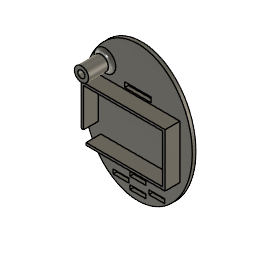
Panel2 (Autodesk Fusion 360 design; units mm, degrees)
part number: 2026-05-24-13-53-39-480
Autodesk Fusion 360 part; units mm, degrees
sketch "Sketch1" plane through (0, 0, 0) normal (0, 1, 0) x (1, 0, 0)
  ellipse E0 centre (0, 0) end of major axis (0, 27.5) minor radius 22
  line L0 (0, -27.5) -> (0, 27.5) construction
  line L1 (22, 0) -> (-22, 0) construction
  dimension "d1" = 44
  dimension "d2" = 55
  constraint coincident E0 L0.start
  constraint coincident E0 L0.end
  constraint coincident E0 L1.start
  constraint coincident E0 L1.end
  constraint coincident E0.centre origin
  constraint vertical L0
  measures "d2" distance of E0
extrude "Extrude1" add sketch "Sketch1" along normal blind 1.5
sketch "Sketch2" plane through (0, 0, 0) normal (0, -1, 0) x (1, 0, 0)
  ellipse E0 centre (0, 0) end of major axis (0, -27.5) minor radius 22
  line L0 (-5.35, 11.5) -> (5.35, 11.5)
  line L1 (5.35, 11.5) -> (5.35, 9.5)
  line L2 (5.35, 9.5) -> (-5.35, 9.5)
  line L3 (-5.35, 9.5) -> (-5.35, 11.5)
  point P0 (0, 27.5)
  dimension "d5" = 10.7
  dimension "d6" = 2
  dimension "d7" = 16
  constraint horizontal L0
  constraint vertical L1
  constraint horizontal L2
  constraint vertical L3
  constraint coincident E0 P0
  measures "d5" distance of L1.end L2.end
  measures "d6" distance of L0.start L2.end
  measures "d7" distance of L0 P0
extrude "Extrude2" cut sketch "Sketch2" against normal blind 10 contours L0 L1 L2 L3
sketch "Sketch3" plane through (0, 0, 0) normal (0, -1, 0) x (1, 0, 0)
  line L0 (5.35, 11.5) -> (5.35, 9.5)
  line L1 (5.35, 9.5) -> (-5.35, 9.5)
  line L2 (-5.35, 9.5) -> (-5.35, 11.5)
  line L3 (-5.35, 11.5) -> (5.35, 11.5)
  ellipse E0 centre (0, 0) end of major axis (0, -27.5) minor radius 22
  circle A0 centre (-13.3446, 14.9401) radius 1.45
  circle A1 centre (-13.3446, 14.9401) radius 2.9
  dimension "d10" = 2.9
  dimension "d11" = 5.8
  constraint concentric A0 A1
  measures "d10" diameter of A0
  measures "d11" diameter of A1
extrude "Extrude3" add sketch "Sketch3" along normal blind 9.5 contours A1
fillet "Fillet1" radius 1.5 1 edges at (-16.0483, 0, 15.9888)
sketch "Sketch4" plane through (0, 0, 0) normal (0, -1, 0) x (1, 0, 0)
  line L0 (5.35, 11.5) -> (5.35, 9.5)
  line L1 (5.35, 9.5) -> (-5.35, 9.5)
  line L2 (-5.35, 9.5) -> (-5.35, 11.5)
  line L3 (-5.35, 11.5) -> (5.35, 11.5)
  line L4 (-16, 7.9) -> (16, 7.9)
  line L5 (16, 7.9) -> (16, -11.6)
  line L6 (16, -11.6) -> (-16, -11.6)
  line L7 (-16, -11.6) -> (-16, 7.9)
  line L8 (-17, 8.9) -> (17, 8.9)
  line L9 (17, 8.9) -> (17, -12.6)
  line L10 (17, -12.6) -> (-17, -12.6)
  line L11 (-17, -12.6) -> (-17, 8.9)
  ellipse E0 centre (0, 0) end of major axis (0, -27.5) minor radius 22
  circle A0 centre (-13.3446, 14.9401) radius 4.4
  dimension "d16" = 32
  dimension "d17" = 19.5
  dimension "d18" = 1
  dimension "d19" = 1
  dimension "d20" = 1
  dimension "d21" = 1
  dimension "d22" = 0.6
  constraint horizontal L4
  constraint vertical L5
  constraint horizontal L6
  constraint vertical L7
  constraint horizontal L8
  constraint vertical L9
  constraint horizontal L10
  constraint vertical L11
  measures "d16" distance of L4.start L4.end
  measures "d17" distance of L4.start L6.end
  measures "d18" distance of L6 L10
  measures "d19" distance of L5 L9
  measures "d20" distance of L4 L8
  measures "d21" distance of L7 L11
  measures "d22" distance of L1 L8
extrude "Extrude4" add sketch "Sketch4" along normal blind 6 contours L8 L9 L10 L11
sketch "Sketch5" plane through (0, 0, 0) normal (0, -1, 0) x (1, 0, 0)
  circle A0 centre (-13.3446, 14.9401) radius 4.4
  ellipse E0 centre (0, 0) end of major axis (0, -27.5) minor radius 22
  line L0 (5.35, 11.5) -> (5.35, 9.5)
  line L1 (5.35, 9.5) -> (-5.35, 9.5)
  line L2 (-5.35, 9.5) -> (-5.35, 11.5)
  line L3 (-5.35, 11.5) -> (5.35, 11.5)
  line L4 (-17, -12.6) -> (-17, 8.9)
  line L5 (-17, 8.9) -> (17, 8.9)
  line L6 (17, 8.9) -> (17, -12.6)
  line L7 (17, -12.6) -> (-17, -12.6)
  line L8 (-17, -7.6621) -> (-15, -7.6621)
  line L9 (-15, -7.6621) -> (-15, -12.6621)
  line L10 (-15, -12.6621) -> (-17, -12.6621)
  line L11 (-17, -12.6621) -> (-17, -7.6621)
  dimension "d25" = 2
  dimension "d26" = 5
  constraint horizontal L8
  constraint vertical L9
  constraint horizontal L10
  constraint vertical L11
  constraint coincident L4 L8.start
  measures "d25" distance of L8.start L8.end
  measures "d26" distance of L8.start L10.end
extrude "Extrude5" cut sketch "Sketch5" along normal blind 6.8 contours L4 L7 L8 L9 L11 | L7 L9 L10 L11
sketch "Sketch6" plane through (0, 0, 0) normal (0, -1, 0) x (1, 0, 0)
  line L0 (5.35, 11.5) -> (5.35, 9.5)
  line L1 (5.35, 9.5) -> (-5.35, 9.5)
  line L2 (-5.35, 9.5) -> (-5.35, 11.5)
  line L3 (-5.35, 11.5) -> (5.35, 11.5)
  ellipse E0 centre (0, 0) end of major axis (0, -27.5) minor radius 22
  circle A0 centre (-13.3446, 14.9401) radius 4.4
  line L4 (-16, -7.6621) -> (-17, -7.6621)
  line L5 (-17, -7.6621) -> (-17, 8.9)
  line L6 (-17, 8.9) -> (17, 8.9)
  line L7 (17, 8.9) -> (17, -12.6)
  line L8 (17, -12.6) -> (-15, -12.6)
  line L9 (-15, -12.6) -> (-15, -11.6)
  line L10 (-15, -11.6) -> (16, -11.6)
  line L11 (16, -11.6) -> (16, 7.9)
  line L12 (16, 7.9) -> (-16, 7.9)
  line L13 (-16, 7.9) -> (-16, -7.6621)
  line L14 (4.4492, -16.8) -> (10.8492, -16.8)
  line L15 (10.8492, -16.8) -> (10.8492, -18.5)
  line L16 (10.8492, -18.5) -> (4.4492, -18.5)
  line L17 (4.4492, -18.5) -> (4.4492, -16.8)
  line L18 (-15, -12.6) -> (17, -12.6)
  line L19 (-9.9508, -16.8) -> (-3.5508, -16.8)
  line L20 (-3.5508, -16.8) -> (-3.5508, -18.5)
  line L21 (-3.5508, -18.5) -> (-9.9508, -18.5)
  line L22 (-9.9508, -18.5) -> (-9.9508, -16.8)
  line L23 (-3.2, -18.8) -> (3.2, -18.8)
  line L24 (3.2, -18.8) -> (3.2, -20.5)
  line L25 (3.2, -20.5) -> (-3.2, -20.5)
  line L26 (-3.2, -20.5) -> (-3.2, -18.8)
  line L27 (-10.0508, -21.4) -> (-3.6508, -21.4)
  line L28 (-3.6508, -21.4) -> (-3.6508, -23.1)
  line L29 (-3.6508, -23.1) -> (-10.0508, -23.1)
  line L30 (-10.0508, -23.1) -> (-10.0508, -21.4)
  line L31 (4.4492, -21.4) -> (10.8492, -21.4)
  line L32 (10.8492, -21.4) -> (10.8492, -23.1)
  line L33 (10.8492, -23.1) -> (4.4492, -23.1)
  line L34 (4.4492, -23.1) -> (4.4492, -21.4)
  line L35 (-3.2, -23.5) -> (3.2, -23.5)
  line L36 (3.2, -23.5) -> (3.2, -25.2)
  line L37 (3.2, -25.2) -> (-3.2, -25.2)
  line L38 (-3.2, -25.2) -> (-3.2, -23.5)
  dimension "d29" = 6.4
  dimension "d30" = 1.7
  dimension "d31" = 4.2
  dimension "d32" = 6.4
  dimension "d33" = 1.7
  dimension "d34" = 8
  dimension "d35" = 4.2
  dimension "d36" = 6.4
  dimension "d37" = 1.7
  dimension "d38" = 6.2
  dimension "d39" = 6.4
  dimension "d40" = 1.7
  dimension "d41" = 8.8
  dimension "d42" = 6.4
  dimension "d43" = 1.7
  dimension "d44" = 8.8
  dimension "d45" = 8.1
  dimension "d46" = 6.4
  dimension "d47" = 1.7
  dimension "d48" = 10.9
  constraint horizontal L14
  constraint vertical L15
  constraint horizontal L16
  constraint vertical L17
  constraint horizontal L19
  constraint vertical L20
  constraint horizontal L21
  constraint vertical L22
  constraint horizontal L23
  constraint vertical L24
  constraint horizontal L25
  constraint vertical L26
  constraint horizontal L27
  constraint vertical L28
  constraint horizontal L29
  constraint vertical L30
  constraint horizontal L31
  constraint vertical L32
  constraint horizontal L33
  constraint vertical L34
  constraint collinear L17 L34
  constraint horizontal L35
  constraint vertical L36
  constraint horizontal L37
  constraint vertical L38
  constraint collinear L26 L38
  measures "d29" distance of L14.start L14.end
  measures "d30" distance of L14.start L16.end
  measures "d31" distance of L14 L18
  measures "d32" distance of L19.start L19.end
  measures "d33" distance of L19.start L21.end
  measures "d34" distance of L17 L20
  measures "d35" distance of L18 L19
  measures "d36" distance of L23.start L23.end
  measures "d37" distance of L23.start L25.end
  measures "d38" distance of L18 L23
  measures "d39" distance of L27.start L27.end
  measures "d40" distance of L27.start L29.end
  measures "d41" distance of L18 L27
  measures "d42" distance of L31.start L31.end
  measures "d43" distance of L31.start L33.end
  measures "d44" distance of L18 L31
  measures "d45" distance of L28 L34
  measures "d46" distance of L35.start L35.end
  measures "d47" distance of L35.start L37.end
  measures "d48" distance of L18 L35
extrude "Extrude6" cut sketch "Sketch6" against normal blind 5 contours L14 L15 L16 L17 | L19 L20 L21 L22 | L23 L24 L25 L26 | L27 L28 L29 L30 | L31 L32 L33 L34 | L35 L36 L37 L38
